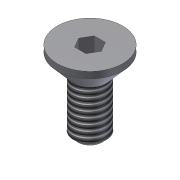
# Autodesk Inventor part: Part8
Saved by Autodesk Inventor 2011 (Build 150239000, 239)
## iProperties
Created: 2012-04-06
Part Number: Part8
Document SubType Name: Modeling
Designer: jhanson2
Density: 1 g/cm^3
Author: jhanson2
Autodesk Inventor part; units mm, degrees
ref_plane "YZ Plane" through (0, 0, 0) normal (1, 0, 0) x (0, 1, 0)
ref_plane "XZ Plane" through (0, 0, 0) normal (0, 1, 0) x (-1, 0, 0)
ref_plane "XY Plane" through (0, 0, 0) normal (0, 0, 1) x (1, 0, 0)
sketch "Sketch1" plane through (0, 0, 0) normal (0, 0, 1) x (1, 0, 0)
  line L0 (0, 0) -> (-7.9375, 0)
  line L1 (-7.9375, 0) -> (-7.9375, -1.5875)
  line L2 (-7.9375, -1.5875) -> (-3.9687, -6.153)
  line L3 (-3.9687, -6.153) -> (-3.9687, -19.05)
  line L4 (-3.9687, -19.05) -> (0, -19.05)
  line L5 (0, -19.05) -> (0, 0)
  dimension "d0" = 15.875
  dimension "d1" = 1.5875
  dimension "d2" = 19.05
  dimension "d3" = 7.9375
  dimension "d16" = 41
  constraints: 12 end point, 3 parallel, 1 horizontal, 1 perpendicular
  measures "d0" diameter of L0.end L5
  measures "d1" distance of L1.end L0.end
  measures "d2" distance from line of L3.end L0
  measures "d3" diameter of L3 L5
  measures "d16" angle of L5 L2
revolve "Revolution1" add sketch "Sketch1" angle 360 about axis through (0, -19.05, 0) along (0, 1, 0)
chamfer "Chamfer1" distance 1.016 angle 45 1 edges at (3.9688, -19.05, 0)
thread "Thread1" size "5/16-18 UNC" class "2A" standard "ANSI Unified Screw Threads" full length
sketch "Sketch2" plane through (0, 0, 0) normal (0, 1, 0) x (1, 0, 0)
  circle A0 centre (0, 0) radius 7.9375 projected
  line L0 (-1.3748, -2.3812) -> (-2.7496, 0)
  line L1 (-2.7496, 0) -> (-1.3748, 2.3813)
  line L2 (-1.3748, 2.3813) -> (1.3748, 2.3813)
  line L3 (1.3748, 2.3813) -> (2.7496, 0)
  line L4 (2.7496, 0) -> (1.3748, -2.3813)
  line L5 (1.3748, -2.3813) -> (-1.3748, -2.3812)
  dimension "d11" = 4.7625
  constraints: 12 end point, 1 coincident, 1 horizontal, 13 other
  measures "d11" distance between parallel lines of L4 L1
extrude "Extrusion1" cut sketch "Sketch2" against normal blind 3.429 contours L0 L1 L2 L3 L4 L5
sketch "Sketch3" plane through (0, -3.429, 0) normal (0, 1, 0) x (1, 0, 0)
  line L0 (-1.3748, -2.3812) -> (1.3748, -2.3813) projected
  line L1 (1.3748, -2.3813) -> (2.7496, 0) projected
  line L2 (2.7496, 0) -> (1.3748, 2.3813) projected
  line L3 (1.3748, 2.3813) -> (-1.3748, 2.3813) projected
  line L4 (-1.3748, 2.3813) -> (-2.7496, 0) projected
  line L5 (-2.7496, 0) -> (-1.3748, -2.3812) projected
  point P0 (0, 0)
extrude "Extrusion2" cut sketch "Sketch3" against normal blind 0.254 draft -83
body "Solid1"
